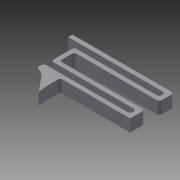
# Autodesk Inventor part: ValveRatcheKeep
Saved by Autodesk Inventor 2015 (Build 190159000, 159)
## iProperties
Created: 2016-01-09
Part Number: ValveRatcheKeep
Material: Generic
Document SubType Name: Modeling
Designer: HP USER
Density: 1 g/cm^3
Appearance: Default
Author: HP USER
Autodesk Inventor part; units mm, degrees
ref_plane "YZ Plane" through (0, 0, 0) normal (1, 0, 0) x (0, 1, 0)
ref_plane "XZ Plane" through (0, 0, 0) normal (0, 1, 0) x (-1, 0, 0)
ref_plane "XY Plane" through (0, 0, 0) normal (0, 0, 1) x (1, 0, 0)
sketch "Sketch1" plane through (0, 0, 0) normal (0, 0, 1) x (1, 0, 0)
  line L0 (1.1222, 11.6795) -> (12.6128, 11.6795)
  line L1 (12.6128, 11.6795) -> (12.6128, 14.0795)
  line L2 (12.6128, 14.0795) -> (-1.3872, 14.0795)
  line L3 (-1.3872, 14.0795) -> (-1.3872, 16.4795)
  line L4 (-1.3872, 16.4795) -> (12.6128, 16.4795)
  line L5 (12.6128, 16.4795) -> (12.6128, 18.8795)
  line L6 (12.6128, 18.8795) -> (-2.0872, 18.8795)
  line L7 (-2.3189, 12.3795) -> (11.9128, 12.3795)
  line L8 (11.9128, 12.3795) -> (11.9128, 13.3795)
  line L9 (11.9128, 13.3795) -> (-2.0872, 13.3795)
  line L10 (-2.0872, 13.3795) -> (-2.0872, 17.1795)
  line L11 (-2.0872, 17.1795) -> (11.9128, 17.1795)
  line L12 (11.9128, 17.1795) -> (11.9128, 18.1795)
  line L13 (11.9128, 18.1795) -> (-2.0872, 18.1795)
  line L14 (-2.0872, 18.1795) -> (-2.0872, 18.8795)
  line L15 (-2.0872, 17.1795) -> (11.9128, 17.1795)
  line L16 (11.9128, 17.1795) -> (11.9128, 18.1795)
  line L17 (11.9128, 18.1795) -> (-2.0872, 18.1795)
  line L18 (-2.0872, 18.1795) -> (-2.0872, 18.8795)
  line L19 (-2.0872, 18.8795) -> (12.6128, 18.8795)
  line L20 (12.6128, 18.8795) -> (12.6128, 16.4795)
  line L21 (12.6128, 16.4795) -> (-1.3872, 16.4795)
  line L22 (-1.3872, 16.4795) -> (-1.3872, 14.0795)
  line L23 (-1.3872, 14.0795) -> (12.6128, 14.0795)
  line L24 (12.6128, 14.0795) -> (12.6128, 11.6795)
  line L25 (1.1222, 11.6795) -> (1.1222, 9.8639)
  line L26 (1.1222, 9.8639) -> (1.2928, 7.9819)
  line L27 (1.2928, 7.9819) -> (-1.4976, 11.3795)
  line L28 (-2.3189, 12.3795) -> (-2.3189, 11.3795)
  line L29 (-2.3189, 11.3795) -> (-1.4976, 11.3795)
  dimension "d3" = 2.4
  dimension "d4" = 14
  dimension "d5" = 2.4
  dimension "d6" = 2.4
  dimension "d9" = 1
  dimension "d10" = 14
  dimension "d11" = 3.8
  dimension "d12" = 1
  dimension "d24" = 1
  constraints: 60 end point, 12 perpendicular, 4 point on line, 2 vertical, 1 parallel, 9 other
  measures "d3" distance of L0.end L1.end
  measures "d4" distance of L1.end L2.end
  measures "d5" distance of L2.end L3.end
  measures "d6" distance of L4.end L5.end
  measures "d9" distance of L7.end L8.end
  measures "d10" distance of L8.end L9.end
  measures "d11" distance of L9.end L10.end
  measures "d12" distance of L11.end L12.end
  measures "d24" distance of L7.start L28.end
extrude "Extrusion1" add sketch "Sketch1" along normal blind 2
fillet "Fillet1" radius 0.4 13 edges at (-1.3872, 14.0795, 1) (-1.3872, 16.4795, 1) (-2.0872, 13.3795, 1) (-2.0872, 17.1795, 1) (11.9128, 13.3795, 1) (11.9128, 12.3795, 1) (12.6128, 14.0795, 1) (12.6128, 16.4795, 1) (11.9128, 17.1795, 1) (11.9128, 18.1795, 1) (12.6128, 18.8795, 1) (1.1222, 11.6795, 1) (-2.3189, 12.3795, 1)
sketch "Sketch2" plane through (-2.0872, 18.1795, 0) normal (-1, 0, 0) x (0, 0, 1)
  line L0 (0, 0.7) -> (0, 0) projected
  line L1 (0, 0) -> (2, 0) projected
  line L2 (2, 0.7) -> (2, 0) projected
  line L3 (0, 0.7) -> (2, 0.7) projected
  point P0 (0, -18.1795)
extrude "Extrusion2" add sketch "Sketch2" along normal blind 2
chamfer "Chamfer1" distance 0.8 angle 45 1 edges at (-1.4976, 11.3795, 1)
body "Solid1"
